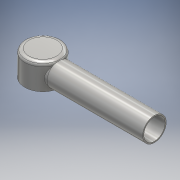
# Autodesk Inventor part: UR5 extended arm
Saved by Autodesk Inventor 2016 (Build 200138000, 138)
## iProperties
Created: 2017-12-24
Part Number: UR5 extended arm
Material: Aluminum 6061-AHC
Document SubType Name: Modeling
Designer: kornbot
Density: 2.7 g/cm^3
Appearance: Aluminum - Dark
Mass: 285.502 g
Surface Area: 950.192 cm^2
Volume: 105.741 cm^3
Author: kornbot
Autodesk Inventor part; units mm, degrees
ref_plane "YZ Plane" through (0, 0, 0) normal (1, 0, 0) x (0, 1, 0)
sketch "Sketch1" plane through (0, 0, 0) normal (0, 0, 1) x (1, 0, 0)
  circle A0 centre (0, 0) radius 38.1195
  circle A1 centre (0, 0) radius 39.6195
  dimension "d0" = 76.239
  dimension "d1" = 79.239
  constraints: 2 centre point, 2 coincident
  measures "d0" diameter of A0
  measures "d1" diameter of A1
extrude "Extrusion1" add sketch "Sketch1" along normal blind 45.75
sketch "Sketch2" plane through (0, 0, 45.75) normal (0, 0, 1) x (1, 0, 0)
  circle A0 centre (0, 0) radius 39.6195
  constraints: 1 centre point, 1 coincident
extrude "Extrusion2" add sketch "Sketch2" along normal blind 9
fillet "Fillet1" radius 7.25 1 edges at (-39.6195, 0, 54.75)
ref_plane "Work Plane33" through (0, 0, 50.25) normal (0, 0, -1) x (-1, 0, 0)
sketch "Sketch3" plane through (0, 0, 50.25) normal (0, 0, -1) x (-1, 0, 0)
  line L0 (-47.3366, 22.9327) -> (-41.452, 22.9327)
  line L1 (-41.452, 22.9327) -> (-41.452, -26.7404)
  line L2 (-41.452, -26.7404) -> (-47.3366, -26.7404)
  line L3 (-47.3366, -26.7404) -> (-47.3366, 22.9327)
  point P0 (0, 0)
  constraints: 8 end point, 2 parallel, 1 horizontal, 1 perpendicular
extrude "Extrusion3" add sketch "Sketch3" along normal blind 50.5
ref_plane "Work Plane17" through (47.3366, -26.7404, 50.25) normal (1, 0, 0) x (0, 0, -1)
sketch "Sketch4" plane through (47.3366, -26.7404, 50.25) normal (1, 0, 0) x (0, 0, -1)
  line L0 (0, 0) -> (0, 49.6732) projected
  line L1 (0, 0) -> (50.25, 51.0864)
  line L2 (50.25, -12.8791) -> (50.25, 66.3599) projected
  line L3 (0, 49.6732) -> (50.5, 49.6732) projected
  line L4 (50.5, 49.6732) -> (50.5, 0) projected
  line L5 (0, 49.6732) -> (50.5, 0)
  circle A0 centre (24.8332, 25.2466) radius 25
  circle A1 centre (24.8332, 25.2466) radius 23.5
  point P0 (50.25, 26.7404)
  dimension "d10" = 50
  dimension "d11" = 47
  constraints: 4 end point, 2 centre point, 1 coincident, 1 perpendicular, 1 point on line
  measures "d10" diameter of A0
  measures "d11" diameter of A1
extrude "Extrusion4" add sketch "Sketch4" along normal blind 200 contours A0 L0 | L0 A0 L5 A1 L1 | L1 A1 L5 A0 | L5 A1 L1 A0 | A0 L3 L1 A1 L5 | A0 L3
ref_plane "Work Plane34" through (41.452, -26.7404, 50.25) normal (0, -1, 0) x (1, 0, 0)
sketch "Sketch5" plane through (41.452, -26.7404, 50.25) normal (0, -1, 0) x (1, 0, 0)
  line L0 (0, 0) -> (5.8846, 0) projected
  line L1 (5.8846, -30.1568) -> (5.8846, -50.5) projected
  line L2 (0, 0) -> (5.8846, 0)
  line L3 (5.8846, 0) -> (5.8846, -50.5)
  line L4 (5.8846, -50.5) -> (0, -50.5)
  line L5 (0, -50.5) -> (0, 0)
  point P0 (-41.452, -50.25)
  constraints: 8 end point, 2 parallel, 1 horizontal, 1 perpendicular
extrude "Extrusion5" cut sketch "Sketch5" against normal blind 173.5
sketch "Sketch6" plane through (247.3366, -1.4939, 25.4168) normal (1, 0, 0) x (0, 0, -1)
  circle A0 centre (0, 0) radius 24.9533
  circle A1 centre (0, 0) radius 23.5
  point P0 (25.4168, 1.4939)
  constraints: 2 centre point, 1 coincident
extrude "Extrusion6" add sketch "Sketch6" against normal blind 218
sketch "Sketch7" plane through (0, 0, 0) normal (0, 0, -1) x (-1, 0, 0)
  arc A0 (-34.6182, -15.9587) -> (-35.8448, 12.9709) centre (0, 0) ccw projected
  line L0 (-29.3366, -24.3405) -> (-29.3366, 23.4595) projected
  line L1 (-29.3366, 24.3405) -> (-29.3366, -24.3405)
  line L2 (-29.3366, 23.4595) -> (-37.7821, 23.4595)
  line L3 (-37.7821, 23.4595) -> (-37.7821, -20.2258)
  line L4 (-37.7821, -20.2258) -> (-29.3366, -20.2258)
  line L5 (-29.3366, -20.2258) -> (-29.3366, 23.4595)
  line L6 (-34.6182, 15.9587) -> (-29.3366, 15.9587)
  line L7 (-29.3366, 15.9587) -> (-29.3366, -15.0516)
  line L8 (-29.3366, -15.0516) -> (-34.6182, -15.0516)
  line L9 (-34.6182, -15.0516) -> (-34.6182, 15.9587)
  point P0 (-29.3366, 12.9709)
  constraints: 18 end point, 4 parallel, 2 horizontal, 2 perpendicular, 2 point on circle, 1 point on line, 1 vertical
extrude "Extrusion7" cut sketch "Sketch7" against normal blind 47.75 contours L8 L9 L6 L0
sketch "Sketch8" plane through (247.3366, -1.4939, 25.4168) normal (1, 0, 0) x (0, 0, -1)
  circle A0 centre (0, 0) radius 23.5
  point P0 (25.4168, 1.4939)
  constraints: 1 centre point
extrude "Extrusion8" cut sketch "Sketch8" against normal blind 258.5
sketch "Sketch9" plane through (0, 0, 54.75) normal (0, 0, 1) x (1, 0, 0)
  circle A0 centre (0, 0) radius 37.5712
  circle A1 centre (0, 0) radius 37.5712
  constraints: 2 centre point, 2 coincident, 1 concentric
extrude "Extrusion9" cut sketch "Sketch9" against normal blind 122
sketch "Sketch10" plane through (0, 0, 45.75) normal (0, 0, -1) x (-1, 0, 0)
  circle A0 centre (0, 0) radius 37.5712
  constraints: 1 centre point, 1 coincident
extrude "Extrusion10" add sketch "Sketch10" against normal blind 9.5
fillet "Fillet2" radius 10.75 1 edges at (37.5712, 0, 55.25)
sketch "Sketch11" plane through (247.3366, -1.4939, 25.4168) normal (1, 0, 0) x (0, 0, -1)
  circle A0 centre (0, 0) radius 26.0768
  circle A1 centre (0, 0) radius 25
  point P0 (25.4168, 1.4939)
  constraints: 2 centre point, 1 coincident
extrude "Extrusion11" add sketch "Sketch11" against normal blind 210.25
body "Solid1"
